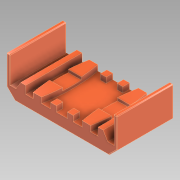
# Autodesk Inventor part: PillarTopVD
Saved by Autodesk Inventor 2021 (Build 250183000, 183)
## iProperties
Created: 2021-03-07
Part Number: PillarTopVD
Material: 一般
Document SubType Name: Modeling
Designer: kumagai
Density: 1 g/cm^3
Appearance: 滑らか - 淡いオレンジ
Author: kumagai
Autodesk Inventor part; units mm, degrees
ref_plane "YZ Plane" through (0, 0, 0) normal (1, 0, 0) x (0, 1, 0)
ref_plane "XZ Plane" through (0, 0, 0) normal (0, 1, 0) x (-1, 0, 0)
ref_plane "XY Plane" through (0, 0, 0) normal (0, 0, 1) x (1, 0, 0)
sketch "スケッチ1" plane through (0, 0, 0) normal (0, 1, 0) x (-1, 0, 0)
  line L0 (0, -21.0065) -> (0, 21.0391) projected
  line L1 (-95.27, 0) -> (121.47, 0) projected
  line L2 (22, -15) -> (-22, -15)
  line L3 (-22, -15) -> (-22, 15)
  line L4 (-22, 15) -> (22, 15)
  line L5 (22, 15) -> (22, -15)
  line L6 (6, 15) -> (2.9, 15)
  line L7 (2.9, 15) -> (2.9, 11.5)
  line L8 (2.9, 11.5) -> (6, 11.5)
  line L9 (6, 11.5) -> (6, 15)
  arc A0 (10.85, 15) -> (9.45, 0) centre (90.5071, 0) ccw
  arc A1 (16.75, 0) -> (15.35, 15) centre (-64.3071, 0) ccw
  line L10 (13.1, -2.0457) -> (13.1, 1.915)
  line L11 (16.75, 0) -> (9.45, 0)
  line L12 (15.35, 15) -> (10.85, 15)
  line L13 (16.5956, 5) -> (9.6044, 5)
  line L14 (19.25, -15) -> (19.25, 15)
  point P0 (0, 0)
  point P1 (2.9, 15)
  point P2 (19.25, 0)
  point P3 (22, 0)
  dimension "d0" = 44
  dimension "d1" = 30
  dimension "d18" = 3.5
  dimension "d19" = 6
  dimension "d20" = 3.1
  dimension "d21" = 16.75
  dimension "d22" = 7.3
  dimension "d25" = 4.5
  dimension "d26" = 10
  dimension "d28" = 6.9913
  dimension "d37" = 2.9
  dimension "d38" = 19.25
  constraints: 26 end point, 7 point on line, 6 point on circle, 5 parallel, 4 horizontal, 3 perpendicular, 2 centre point, 1 line through centre, 1 vertical, 3 other
  measures "d0" distance between parallel lines of L3 L5
  measures "d1" distance between parallel lines of L4 L2
  measures "d18" distance between parallel lines of L4 L8
  measures "d19" distance between parallel lines of L9 L0
  measures "d20" distance between parallel lines of L9 L7
  measures "d21" distance from line of L11.start L0
  measures "d22" distance of L11.start L11.end
  measures "d25" distance of L12.end L12.start
  measures "d26" distance between parallel lines of L4 L13
  measures "d28" distance of L13.start L13.end
  measures "d37" distance between parallel lines of L7 L0
  measures "d38" distance between parallel lines of L14 L0
extrude "押し出し1" add sketch "スケッチ1" against normal blind 2
extrude "押し出し3" add sketch "スケッチ1" along normal blind 3 contours L4 L9 L8 L7 | A0 L4 A1 L13
extrude "押し出し4" add sketch "スケッチ1" along normal blind 1.5 contours A0 L13 A1 L1
mirror "ミラー1" about plane through (0, 0, 0) normal (0, 0, 1) of "押し出し1", "押し出し3", "押し出し4"
extrude "押し出し5" add sketch "スケッチ1" along normal blind 4.2 contours L14 L1 L5 L2 | L14 L4 L5 L1
mirror "ミラー3" about plane through (0, 0, 0) normal (1, 0, 0) of "押し出し1", "押し出し3", "押し出し4", "ミラー1", "押し出し5"
sketch "スケッチ2" plane through (0, 0, 0) normal (0, 0, 1) x (1, 0, 0)
  line L0 (0, 5.44) -> (0, -3.24) projected
  line L1 (-30.8, 0) -> (30.8, 0) projected
  line L2 (-29.5, 14.3) -> (-27.5, 14.3)
  line L3 (-27.5, 14.3) -> (-27.5, 0)
  line L4 (27.5, 0) -> (27.5, 14.3)
  line L5 (27.5, 14.3) -> (29.5, 14.3)
  line L6 (29.5, 14.3) -> (29.5, -1.4)
  line L7 (29.5, -1.4) -> (25, -5.9)
  line L8 (25, -5.9) -> (-25, -5.9)
  line L9 (-25, -5.9) -> (-29.5, -1.4)
  line L10 (-29.5, -1.4) -> (-29.5, 14.3)
  line L11 (-19.25, 4.2) -> (-22, 4.2) projected
  line L12 (19.25, 4.2) -> (22, 4.2) projected
  line L13 (-22, -2) -> (-22, 4.2) projected
  line L14 (-22, 0) -> (-22, 4.2)
  line L15 (-22, 4.2) -> (-24.4249, 0)
  line L16 (22, -2) -> (22, 4.2) projected
  line L17 (22, 0) -> (22, 4.2)
  line L18 (22, 4.2) -> (24.4249, 0)
  line L19 (-27.5, 0) -> (-24.4249, 0)
  line L20 (-22, 0) -> (22, 0)
  line L21 (24.4249, 0) -> (27.5, 0)
  point P0 (0, 0)
  point P1 (24.4249, 0)
  point P2 (22, 0)
  point P3 (-22, 0)
  point P4 (-24.4249, 0)
  dimension "d41" = 59
  dimension "d42" = 2
  dimension "d44" = 20.2
  dimension "d45" = 45
  dimension "d46" = 50
  dimension "d47" = 120
  dimension "d50" = 14.3
  constraints: 32 end point, 6 point on line, 5 parallel, 3 collinear, 2 perpendicular, 1 horizontal, 4 other
  measures "d41" distance between parallel lines of L6 L10
  measures "d42" distance between parallel lines of L10 L3
  measures "d44" distance between parallel lines of L8 L2
  measures "d45" angle of L8 L9
  measures "d46" distance of L7.end L8.end
  measures "d47" angle of L1 L15
  measures "d50" distance between parallel lines of L2 L1
extrude "押し出し6" add sketch "スケッチ2" along normal mid plane 30
chamfer "面取り1" distance 0.4 angle 45 22 edges at (-29.5, 6.45, 15) (-28.5, 14.3, 15) (-27.5, 7.15, 15) (-27.25, -3.65, 15) (0, -5.9, 15) (27.25, -3.65, 15) (29.5, 6.45, 15) (28.5, 14.3, 15) (27.5, 7.15, 15) (-29.5, 6.45, -15) (-28.5, 14.3, -15) (-27.5, 7.15, -15) (-27.25, -3.65, -15) (0, -5.9, -15) (27.25, -3.65, -15) (29.5, 6.45, -15) (28.5, 14.3, -15) (27.5, 7.15, -15) (-29.5, 14.3, 0) (-27.5, 14.3, 0) (27.5, 14.3, 0) (29.5, 14.3, 0)
equation "\"d39\" = 0.5 * RailHeight"
equation "\"RailHeight\" = 8.4"
